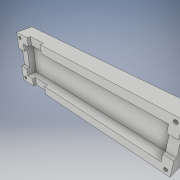
# Autodesk Inventor part: PassiveSwitchCase
Saved by Autodesk Inventor 2019 (Build 230136000, 136)
## iProperties
Created: 2019-05-08
Part Number: PassiveSwitchCase
Material: Generic
Document SubType Name: Modeling
Designer: Tijs
Density: 1 g/cm^3
Appearance: Default
Author: Tijs
Autodesk Inventor part; units mm, degrees
ref_plane "YZ Plane" through (0, 0, 0) normal (1, 0, 0) x (0, 1, 0)
ref_plane "XZ Plane" through (0, 0, 0) normal (0, 1, 0) x (-1, 0, 0)
ref_plane "XY Plane" through (0, 0, 0) normal (0, 0, 1) x (1, 0, 0)
sketch "Sketch1" plane through (0, 0, 0) normal (0, 0, 1) x (1, 0, 0)
  line L0 (-50, -15) -> (50, -15)
  line L1 (50, -15) -> (50, 15)
  line L2 (50, 15) -> (-50, 15)
  line L3 (-50, 15) -> (-50, -15)
  line L4 (-50, -15) -> (50, 15) construction
  line L5 (50, -15) -> (-50, 15) construction
  point P0 (0, 0)
  dimension "d0" = 100
  dimension "d1" = 30
  constraints: 12 end point, 2 midpoint, 2 parallel, 1 horizontal, 1 perpendicular
  measures "d0" distance of L2.end L1.end
  measures "d1" distance of L1.end L0.end
extrude "Extrusion1" add sketch "Sketch1" along normal blind 10
sketch "Sketch2" plane through (0, 0, 10) normal (0, 0, 1) x (1, 0, 0)
  line L0 (-50, -15) -> (50, -15) projected
  line L1 (50, -15) -> (50, 15) projected
  line L2 (50, 15) -> (-50, 15) projected
  line L3 (-50, 15) -> (-50, -15) projected
  line L4 (-45, 10) -> (45, 10)
  line L5 (45, 10) -> (45, -10)
  line L6 (45, -10) -> (-45, -10)
  line L7 (-45, -10) -> (-45, 10)
  point P0 (0, 0)
  dimension "d4" = 5
  constraints: 8 end point, 3 other
  measures "d4" distance between parallel lines of L2 L4
extrude "Extrusion2" cut sketch "Sketch2" against normal blind 6 contours L4 L5 L6 L7
sketch "Sketch3" plane through (0, 0, 10) normal (0, 0, 1) x (1, 0, 0)
  line L0 (-45, -10) -> (-45, 10) projected
  line L1 (-45, 10) -> (45, 10) projected
  line L2 (45, 10) -> (45, -10) projected
  line L3 (45, -10) -> (-45, -10) projected
  line L4 (-50, -15) -> (50, -15) projected
  line L5 (50, -15) -> (50, 15) projected
  line L6 (50, 15) -> (-50, 15) projected
  line L7 (-50, 15) -> (-50, -15) projected
  line L8 (-50, 15) -> (-50, -15) projected
  line L9 (-50, -5.5) -> (-45, -5.5)
  line L10 (-45, -5.5) -> (-45, 5.5)
  line L11 (-45, 5.5) -> (-50, 5.5)
  line L12 (-50, 5.5) -> (-50, -5.5)
  line L13 (-70, 0) -> (70, 0) projected
  line L14 (45, 10) -> (45, -10) projected
  line L15 (50, -15) -> (50, 15) projected
  line L16 (50, 15) -> (-50, 15) projected
  line L17 (-45, 10) -> (45, 10) projected
  line L18 (-40.5, 15) -> (-29.5, 15)
  line L19 (-29.5, 15) -> (-29.5, 10)
  line L20 (-29.5, 10) -> (-40.5, 10)
  line L21 (-40.5, 10) -> (-40.5, 15)
  line L22 (-35, 15) -> (-35, 10) construction
  line L23 (-45, 10) -> (45, 10) projected
  line L24 (45, -10) -> (-45, -10) projected
  line L25 (-50, -15) -> (50, -15) projected
  line L26 (-40.5, -10) -> (-29.5, -10)
  line L27 (-29.5, -10) -> (-29.5, -15)
  line L28 (-29.5, -15) -> (-40.5, -15)
  line L29 (-40.5, -15) -> (-40.5, -10)
  line L30 (45, 10) -> (45, -10) projected
  line L31 (45, 5.5) -> (50, 5.5)
  line L32 (50, 5.5) -> (50, -5.5)
  line L33 (50, -5.5) -> (45, -5.5)
  line L34 (45, -5.5) -> (45, 5.5)
  point P0 (0, 0)
  dimension "d7" = 11
  dimension "d9" = 11
  dimension "d10" = 15
  dimension "d28" = 11
  dimension "d29" = 11
  constraints: 34 end point, 10 point on line, 9 equal length, 5 perpendicular, 4 horizontal, 2 collinear, 2 other
  measures "d7" distance of L10.end L9.end
  measures "d9" distance of L19.end L20.end
  measures "d10" distance between parallel lines of L7 L22
  measures "d28" distance of L27.end L28.end
  measures "d29" distance between parallel lines of L31 L33
extrude "Extrusion3" cut sketch "Sketch3" against normal blind 2 contours L9 L7 L13 L0 | L3 L27 L4 L29 | L13 L7 L11 L0 | L13 L5 L33 L2 | L2 L31 L5 L13 | L21 L6 L19 L1
sketch "Sketch4" plane through (0, 0, 10) normal (0, 0, 1) x (1, 0, 0)
  line L0 (-50, -15) -> (50, -15) projected
  line L1 (-50, 15) -> (-50, -15) projected
  line L2 (50, 15) -> (-50, 15) projected
  line L3 (50, -15) -> (50, 15) projected
  point P0 (0, 0)
  point P1 (-47.5, 12.5)
  dimension "d16" = 2.5
  dimension "d17" = 2.5
  measures "d16" distance from line of L2 point (-47.5, 12.5)
  measures "d17" distance from line of L1 point (-47.5, 12.5)
hole "Hole1" at (-47.5, 12.5, 10) direction (0, 0, -1) diameter 2.013 end through all thread size "M2.5x0.45" class "6H" standard "ANSI Metric M Profile"
mirror "Mirror1" about plane through (0, 0, 0) normal (0, 1, 0) of "Hole1"
mirror "Mirror2" about plane through (0, 0, 0) normal (1, 0, 0) of "Hole1", "Mirror1"
equation "\"d9\" = d7"
equation "\"d28\" = d7"
equation "\"d29\" = d7"
body "Solid1"
